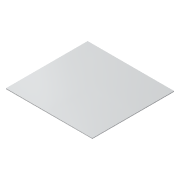
# Autodesk Inventor part: Деталь133
Saved by Autodesk Inventor 2017 (Build 210142000, 142)
## iProperties
Created: 2018-07-04
Part Number: Деталь133
Material: Стекло
Document SubType Name: Sheet Metal
Designer: Евтушенко
Mass: 6256.27 g
Surface Area: 5387.28 cm^2
Volume: 796.978 cm^3
Density: 2.18 g/cm^3
Sheet Metal Rule: По умолчанию_мм
Appearance: Бесцветный
Author: Евтушенко
Autodesk Inventor part; units mm, degrees
ref_plane "YZ Plane" through (0, 0, 0) normal (1, 0, 0) x (0, 1, 0)
ref_plane "XZ Plane" through (0, 0, 0) normal (0, 1, 0) x (-1, 0, 0)
ref_plane "XY Plane" through (0, 0, 0) normal (0, 0, 1) x (1, 0, 0)
sketch "Эскиз5" plane through (0, 0, 0) normal (0, 0, 1) x (1, 0, 0)
  line L0 (-230, -217.5) -> (230, -217.5)
  line L1 (230, -217.5) -> (230, 217.5)
  line L2 (230, 217.5) -> (-230, 217.5)
  line L3 (-230, 217.5) -> (-230, -217.5)
  line L4 (-230, -217.5) -> (230, 217.5) construction
  line L5 (230, -217.5) -> (-230, 217.5) construction
  point P0 (0, 0)
  dimension "d64" = 460
  dimension "d65" = 435
  measures "d64" distance of L2.end L1.end
  measures "d65" distance of L1.end L0.end
extrude "Пластина2" add sketch "Эскиз5" along normal blind 4
equation "\"Радиус_гибки\" = Толщина"
equation "\"Ширина_просечки\" = Толщина"
equation "\"Глубина_просечки\" = 0.5 * Толщина"
equation "\"Размер_высечки\" = 4 * Толщина"
equation "\"Минимальный_остаток\" = 2 * Толщина"
equation "\"Радиус_перехода\" = Радиус_гибки"
equation "\"Радиус_Якоби\" = Радиус_гибки"
equation "\"Размер_зазора\" = Толщина"
equation "\"d2\" = Радиус_гибки"
equation "\"d66\" = Радиус_гибки"
equation "\"Толщина\" = 4"
